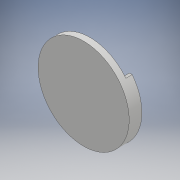
# Autodesk Inventor part: EndCap
Saved by Autodesk Inventor 2018 (Build 220112000, 112)
## iProperties
Created: 2018-05-20
Part Number: EndCap
Material: Generic
Document SubType Name: Modeling
Designer: a
Density: 1 g/cm^3
Appearance: Default
Author: a
Autodesk Inventor part; units mm, degrees
ref_plane "YZ Plane" through (0, 0, 0) normal (1, 0, 0) x (0, 1, 0)
ref_plane "XZ Plane" through (0, 0, 0) normal (0, 1, 0) x (-1, 0, 0)
ref_plane "XY Plane" through (0, 0, 0) normal (0, 0, 1) x (1, 0, 0)
sketch "Sketch1" plane through (0, 0, 0) normal (0, 1, 0) x (-1, 0, 0)
  circle A0 centre (0, 0) radius 21.5
  dimension "d1" = 43
  constraints: 1 centre point
  measures "d1" diameter of A0
extrude "Extrusion1" add sketch "Sketch1" along normal blind 3
sketch "Sketch2" plane through (0, 3, 0) normal (0, 1, 0) x (1, 0, 0)
  arc A0 (15.6228, -13.2732) -> (-15.6228, -13.2732) centre (0, 0) ccw
  arc A1 (16.9137, -13.2732) -> (-16.9137, -13.2732) centre (0, 0) ccw
  circle A2 centre (0, 0) radius 21.5 projected
  line L0 (-16.9137, -13.2732) -> (-15.6228, -13.2732)
  line L1 (15.6228, -13.2732) -> (16.9137, -13.2732)
  dimension "d4" = 41
  constraints: 6 point on circle, 4 end point, 2 centre point, 2 coincident, 2 horizontal
  measures "d4" diameter of A0
extrude "Extrusion2" add sketch "Sketch2" along normal blind 3 contours A0 L0 A1 L1
body "Solid1"
